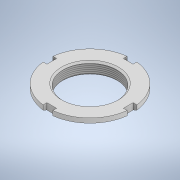
# Autodesk Inventor part: 75. Гайка промежуточного вала
Saved by Autodesk Inventor 2021 (Build 250183000, 183)
## iProperties
Created: 2021-03-15
Part Number: 75. Гайка промежуточного вала
Material: Типовые
Document SubType Name: Modeling
Designer: Данил
Density: 1 g/cm^3
Appearance: По умолчанию
Author: Данил
Autodesk Inventor part; units mm, degrees
ref_plane "YZ Plane" through (0, 0, 0) normal (1, 0, 0) x (0, 1, 0)
ref_plane "XZ Plane" through (0, 0, 0) normal (0, 1, 0) x (-1, 0, 0)
ref_plane "XY Plane" through (0, 0, 0) normal (0, 0, 1) x (1, 0, 0)
sketch "Эскиз1" plane through (0, 0, 0) normal (0, 0, 1) x (1, 0, 0)
  line L0 (0, 3.5) -> (0, -3.5)
  line L1 (17, -3.5) -> (26, 0.6968)
  line L2 (26, 0.6968) -> (26, 3.5)
  line L3 (26, 3.5) -> (17.5, 3.5)
  line L4 (17, -3.5) -> (16.5, -3)
  line L5 (16.5, -3) -> (16.5, 2.5)
  line L6 (0, -3.5) -> (17, -3.5) construction
  line L7 (16.5, 2.5) -> (17.5, 3.5)
  point P0 (0, 0)
  point P1 (0, 0)
  point P2 (16.5, 3.5)
  dimension "d0" = 7
  dimension "d1" = 34
  dimension "d2" = 33
  dimension "d3" = 25
  dimension "d4" = 52
  dimension "d5" = 45
  dimension "d6" = 1
  dimension "d7" = 45
  constraints: 16 end point, 3 vertical, 2 horizontal alignment, 2 point on line, 1 coincident, 1 horizontal, 1 midpoint, 1 perpendicular
  measures "d0" distance of L0.start L0.end
  measures "d1" diameter of L1.start L0
  measures "d2" diameter of L5 L0
  measures "d3" angle of L6 L1
  measures "d4" diameter of L2 L0
  measures "d5" angle of L6 L4
  measures "d6" distance of L5.end point (16.5, 3.5)
  measures "d7" angle of L5 L7
revolve "Вращение1" add sketch "Эскиз1" angle 360 about axis through (0, 3.5, 0) along (0, -1, 0)
sketch "Эскиз2" plane through (0, 3.5, 0) normal (0, 1, 0) x (1, 0, 0)
  line L0 (-3, 26) -> (3, 26)
  line L1 (3, 26) -> (3, 23.5)
  line L2 (3, 23.5) -> (-3, 23.5)
  line L3 (-3, 23.5) -> (-3, 26)
  circle A0 centre (0, 0) radius 26 projected
  point P0 (0, 0)
  point P1 (0, 23.5)
  point P2 (3, 25.8263)
  point P3 (-3, 25.8263)
  dimension "d9" = 6
  dimension "d10" = 2.5
  constraints: 8 end point, 2 parallel, 1 horizontal, 1 midpoint, 1 perpendicular, 1 tangent, 1 vertical alignment
  measures "d9" distance of L1.end L2.end
  measures "d10" distance of L0.end L1.end
extrude "Выдавливание1" cut sketch "Эскиз2" against normal through all contours A0 L1 L2 L3 picked at (0, 24.3333)
pattern_circular "Круговой массив1" count 4 over 360 about axis through (0, 2.0984, 0) along (0, -1, 0) of "Выдавливание1"
thread "Резьба1" size "M33x1" class "6H" standard "ISO Metric profile" length 20
